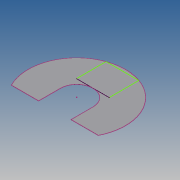
# Autodesk Inventor part: bed
Saved by Autodesk Inventor 2013 (Build 170138000, 138)
## iProperties
Created: 2017-04-12
Part Number: bed
Material: Generic
Document SubType Name: Modeling
Designer: employee
Density: 1 g/cm^3
Author: employee
Autodesk Inventor part; units mm, degrees
ref_plane "YZ Plane" through (0, 0, 0) normal (1, 0, 0) x (0, 1, 0)
ref_plane "XZ Plane" through (0, 0, 0) normal (0, 1, 0) x (-1, 0, 0)
ref_plane "XY Plane" through (0, 0, 0) normal (0, 0, 1) x (1, 0, 0)
sketch "Sketch1" plane through (0, 0, 0) normal (0, 0, 1) x (1, 0, 0)
  arc A0 (100, 0) -> (-100, 0) centre (0, 0) ccw
  arc A1 (267.9086, -135) -> (-267.9086, -135) centre (0, 0) ccw
  line L0 (-100, 0) -> (-100, -135)
  line L1 (-100, -135) -> (-267.9086, -135)
  line L2 (100, 0) -> (100, -135)
  line L3 (100, -135) -> (267.9086, -135)
  dimension "d0" = 200
  dimension "d2" = 600
  dimension "d3" = 135
  constraints: 8 end point, 4 point on circle, 3 perpendicular, 2 centre point, 2 coincident, 2 tangent, 1 parallel, 1 vertical
  measures "d0" diameter of A0
  measures "d2" diameter of A1
  measures "d3" distance of L0.start L0.end
extrude "Extrusion1" add sketch "Sketch1" against normal blind 3
sketch "Sketch2" plane through (0, 0, 0) normal (0, 0, 1) x (1, 0, 0)
  arc A0 (100, 0) -> (-100, 0) centre (0, 0) ccw projected
  line L0 (100, 0) -> (100, -135) projected
  line L1 (100, -135) -> (267.9086, -135) projected
  arc A1 (267.9086, -135) -> (-267.9086, -135) centre (0, 0) ccw projected
  line L2 (-267.9086, -135) -> (-100, -135) projected
  line L3 (-100, -135) -> (-100, 0) projected
  line L4 (-101.709, 282.2327) -> (100, 282.2327)
  line L5 (100, 282.2327) -> (100, 100)
  line L6 (100, 100) -> (-101.709, 100)
  line L7 (-101.709, 100) -> (-101.709, 282.2327)
  constraints: 8 end point, 2 parallel, 1 horizontal, 1 perpendicular, 1 point on circle, 1 tangent
body "Solid1"
